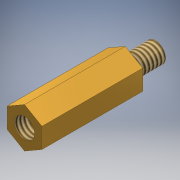
# Autodesk Inventor part: dist5mmM2
Saved by Autodesk Inventor 2016 (Build 200138000, 138)
## iProperties
Created: 2016-09-22
Part Number: dist5mmM2
Material: Brass, Soft Yellow
Document SubType Name: Modeling
Designer: Jakub
Density: 8.47 g/cm^3
Appearance: Brass - Satin
Author: Jakub
Autodesk Inventor part; units mm, degrees
ref_plane "YZ Plane" through (0, 0, 0) normal (1, 0, 0) x (0, 1, 0)
ref_plane "XZ Plane" through (0, 0, 0) normal (0, 1, 0) x (-1, 0, 0)
ref_plane "XY Plane" through (0, 0, 0) normal (0, 0, 1) x (1, 0, 0)
sketch "Sketch1" plane through (0, 0, 0) normal (0, 1, 0) x (-1, 0, 0)
  circle A0 centre (0, 0) radius 1
  line L0 (0, -2) -> (-1.7321, -1)
  line L1 (-1.7321, -1) -> (-1.7321, 1)
  line L2 (-1.7321, 1) -> (0, 2)
  line L3 (0, 2) -> (1.7321, 1)
  line L4 (1.7321, 1) -> (1.7321, -1)
  line L5 (1.7321, -1) -> (0, -2)
  dimension "d0" = 2
  dimension "d1" = 2
  constraints: 12 end point, 2 coincident, 1 centre point, 13 other
  measures "d0" diameter of A0
  measures "d1" distance of L3.end L4.end
extrude "Extrusion1" add sketch "Sketch1" along normal blind 10
sketch "Sketch2" plane through (0, 10, 0) normal (0, 1, 0) x (1, 0, 0)
  circle A0 centre (0, 0) radius 1
  constraints: 1 centre point, 1 coincident
extrude "Extrusion2" add sketch "Sketch2" along normal blind 3
thread "Thread1" size "M2x0.4" class "6g" standard "ANSI Metric M Profile" full length
thread "Thread2" size "M2x0.4" class "6H" standard "ANSI Metric M Profile" full length
body "Solid1"
